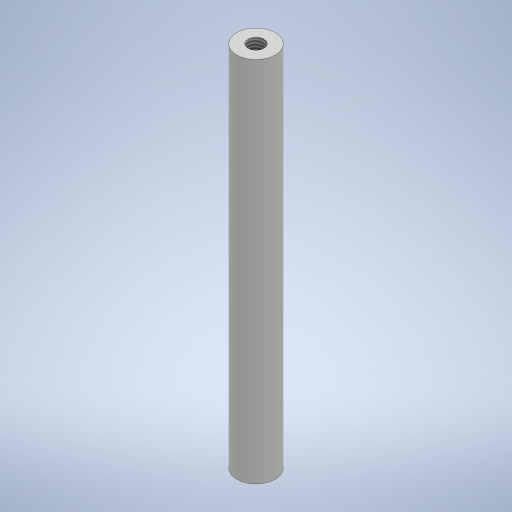
# Autodesk Inventor part: eje
Saved by Autodesk Inventor 2024.2 (Build 282272000, 272)
## iProperties
Created: 2024-11-25
Part Number: eje
Material: Genérico
Document SubType Name: Modeling
Designer: jd.castellanosq
Density: 1 g/cm^3
Appearance: Valor por defecto
Author: jd.castellanosq
Autodesk Inventor part; units mm, degrees
ref_plane "YZ Plane" through (0, 0, 0) normal (1, 0, 0) x (0, 1, 0)
ref_plane "XZ Plane" through (0, 0, 0) normal (0, 1, 0) x (-1, 0, 0)
ref_plane "XY Plane" through (0, 0, 0) normal (0, 0, 1) x (1, 0, 0)
sketch "Boceto1" plane through (0, 0, 0) normal (0, 0, 1) x (1, 0, 0)
  circle A0 centre (0, 0) radius 5
  dimension "d0" = 10
  constraints: 1 centre point, 1 coincident
  measures "d0" diameter of A0
extrude "Extrusión1" add sketch "Boceto1" along normal blind 95
sketch "Boceto2" plane through (0, 0, 95) normal (0, 0, 1) x (1, 0, 0)
  circle A0 centre (0, 0) radius 5 projected
  constraints: 1 coincident
hole "Agujero1" at (0, 0, 95) direction (0, 0, -1) diameter 4.134 depth 15 tip angle 118 thread size "M5x0.8" class "6H" standard "ISO Metric profile"
sketch "Boceto3" plane through (0, 0, 0) normal (0, 0, -1) x (-1, 0, 0)
  point P0 (0, 0)
  point P1 (0, 0)
  constraints: 1 coincident
hole "Agujero2" at (0, 0, 0) direction (0, 0, 1) diameter 4.134 depth 15 tip angle 118 thread size "M5x0.8" class "6H" standard "ISO Metric profile"
